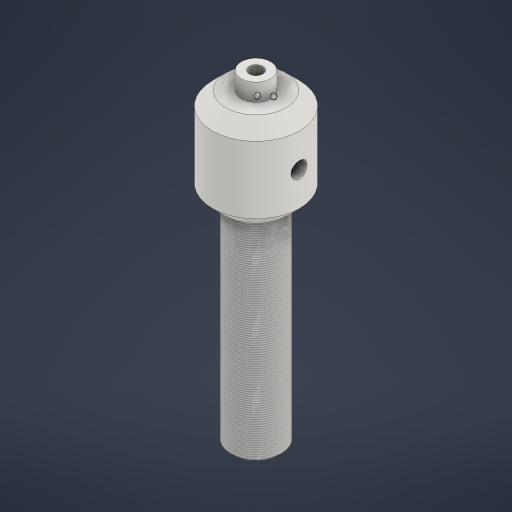
# Autodesk Inventor part: screw.spindle
Saved by Autodesk Inventor 2023 (Build 270158000, 158)
## iProperties
Created: 2023-03-09
Part Number: screw.spindle
Material: Steel, High Strength, Low Alloy
Document SubType Name: Modeling
Designer: kamraj
Density: 7.85 g/cm^3
Appearance: Steel
Author: kamraj
Autodesk Inventor part; units mm, degrees
ref_plane "XZ Plane" through (0, 0, 0) normal (0, 1, 0) x (-1, 0, 0)
ref_plane "XY Plane" through (0, 0, 0) normal (0, 0, 1) x (1, 0, 0)
sketch "Sketch1" plane through (0, 0, 0) normal (0, 1, 0) x (-1, 0, 0)
  circle A0 centre (0, 0) radius 19
  dimension "d0" = 38
  constraints: 1 centre point, 1 coincident
  measures "d0" diameter of A0
extrude "Extrusion1" add sketch "Sketch1" along normal blind 157
sketch "Sketch2" plane through (0, 157, 0) normal (0, 1, 0) x (1, 0, 0)
  circle A0 centre (0, 0) radius 32.5
  dimension "d3" = 65
  constraints: 1 centre point, 1 coincident
  measures "d3" diameter of A0
extrude "Extrusion2" add sketch "Sketch2" along normal blind 70
sketch "Sketch3" plane through (0, 227, 0) normal (0, 1, 0) x (1, 0, 0)
  circle A0 centre (0, 0) radius 11
  dimension "d6" = 22
  constraints: 1 centre point, 1 coincident
  measures "d6" diameter of A0
extrude "Extrusion3" add sketch "Sketch3" along normal blind 13
chamfer "Chamfer1" distance 10 angle 45 2 edges at (-32.5, 227, 0) (-32.5, 157, 0)
chamfer "Chamfer2" distance 2 angle 45 1 edges at (19, 0, 0)
thread "Thread1" size "M38x1.5" class "6g" standard "ISO Metric profile" length 155 offset 3
sketch "Sketch5" plane through (0, 240, 0) normal (0, 1, 0) x (1, 0, 0)
  point P0 (0, 0)
  point P1 (0, 0)
  constraints: 1 coincident
hole "Hole1" at (0, 240, 0) direction (0, -1, 0) diameter 10.106 depth 35 tip angle 118 thread size "M12x1.75" class "6H" standard "ISO Metric profile"
ref_plane "Work Plane1" through (32.5, 157, 0) normal (1, 0, 0) x (0, 1, 0)
sketch "Sketch8" plane through (32.5, 157, 0) normal (1, 0, 0) x (0, 1, 0)
  line L0 (60, -32.5) -> (60, 32.5) projected
  line L1 (10, -32.5) -> (60, -32.5) projected
  line L2 (10, 32.5) -> (10, -32.5) projected
  line L3 (10, 32.5) -> (60, 32.5) projected
  line L4 (60, 32.5) -> (10, -32.5) construction
  line L5 (60, -32.5) -> (10, 32.5) construction
  point P0 (-157, 0)
  point P1 (35, 0)
  constraints: 4 end point, 1 midpoint
hole "Hole3" at (32.5, 192, 0) direction (-1, 0, 0) diameter 12 end through all
